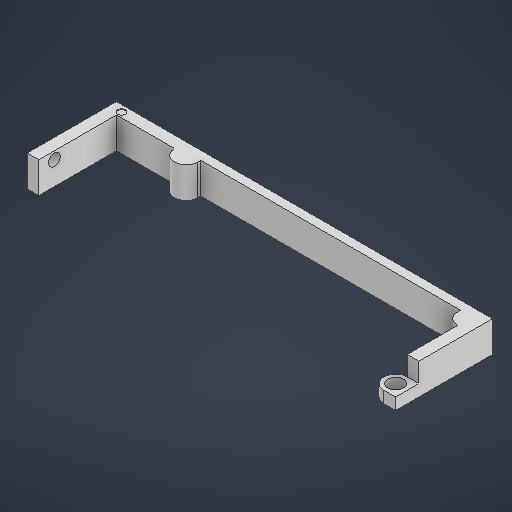
# Autodesk Inventor part: Część4
Saved by Autodesk Inventor 2026.2 (Build 302298010, 298A)
## iProperties
Created: 2026-04-27
Part Number: Część4
Material: Ogólny
Document SubType Name: Modeling
Designer: karol
Density: 1 g/cm^3
Appearance: Domyślna
Author: karol
Autodesk Inventor part; units mm, degrees
ref_plane "YZ Plane" through (0, 0, 0) normal (1, 0, 0) x (0, 1, 0)
ref_plane "XZ Plane" through (0, 0, 0) normal (0, 1, 0) x (-1, 0, 0)
ref_plane "XY Plane" through (0, 0, 0) normal (0, 0, 1) x (1, 0, 0)
sketch "Szkic1" plane through (0, 0, 0) normal (0, 1, 0) x (-1, 0, 0)
  line L0 (0, 0) -> (97, 0)
  line L1 (97, 0) -> (97, -3)
  line L2 (97, -3) -> (0, -3)
  line L3 (0, -3) -> (0, 0)
  dimension "d0" = 97
  dimension "d1" = 3
  constraints: 8 end point, 2 parallel, 1 horizontal, 1 perpendicular
  measures "d0" distance of L1.end L2.end
  measures "d1" distance of L0.end L1.end
extrude "Wyciągnięcie proste1" add sketch "Szkic1" along normal blind 8
sketch "Szkic2" plane through (0, 8, 0) normal (0, 1, 0) x (1, 0, 0)
  circle A0 centre (-94.0035, 1.3347) radius 1
  point P0 (0, 0)
  dimension "d4" = 2
  constraints: 1 centre point
  measures "d4" diameter of A0
extrude "Wyciągnięcie proste2" cut sketch "Szkic2" against normal blind 0.2
sketch "Szkic3" plane through (-97, 0, 0) normal (0, 0, 1) x (1, 0, 0)
  line L0 (97, 8) -> (0, 8) projected
  line L1 (97, 0) -> (94, 0)
  line L2 (94, 0) -> (94, 8)
  line L3 (94, 8) -> (97, 8)
  line L4 (97, 8) -> (97, 0)
  line L5 (0, 0) -> (3, 0)
  line L6 (3, 0) -> (3, 8)
  line L7 (3, 8) -> (0, 8)
  line L8 (0, 8) -> (0, 0)
  dimension "d7" = 3
  dimension "d8" = 3
  constraints: 16 end point, 4 parallel, 3 point on line, 2 horizontal, 2 perpendicular
  measures "d7" distance of L2.end L3.end
  measures "d8" distance of L7.end L6.end
extrude "Wyciągnięcie proste3" add sketch "Szkic3" along normal blind 20 contours L6 L5 L8 L0
extrude "Wyciągnięcie proste4" add sketch "Szkic3" along normal blind 19 contours L4 L1 L2 L0
sketch "Szkic4" plane through (-3, 0, 0) normal (-1, 0, 0) x (0, 0, 1)
  line L0 (19, 8) -> (19, 0) projected
  line L1 (0, 8) -> (19, 8) projected
  line L2 (19, 0) -> (14, 0)
  line L3 (14, 0) -> (14, 8)
  line L4 (14, 8) -> (19, 8)
  line L5 (19, 8) -> (19, 0)
  point P0 (0, 0)
  dimension "d13" = 5
  constraints: 8 end point, 2 parallel, 1 horizontal, 1 perpendicular, 1 point on line
  measures "d13" distance of L3.end L4.end
extrude "Wyciągnięcie proste5" add sketch "Szkic4" along normal blind 3
sketch "Szkic5" plane through (0, 8, 0) normal (0, 1, 0) x (1, 0, 0)
  line L0 (-94, 0) -> (-3, 0) projected
  line L1 (-3, 0) -> (-6, 0)
  line L2 (-6, 0) -> (-6, -3)
  line L3 (-6, -3) -> (-3, -3)
  line L4 (-3, -3) -> (-3, 0)
  line L5 (-79, 0) -> (-73, 0)
  line L6 (-73, 0) -> (-73, -3)
  line L7 (-73, -3) -> (-79, -3)
  line L8 (-79, -3) -> (-79, 0)
  line L9 (-3, 0) -> (-3, -14) projected
  point P0 (0, 0)
  dimension "d16" = 3
  dimension "d17" = 3
  dimension "d18" = 6
  dimension "d19" = 70
  dimension "d20" = 3
  constraints: 16 end point, 4 parallel, 2 horizontal, 2 perpendicular, 2 point on line
  measures "d16" distance of L3.end L2.end
  measures "d17" distance of L2.end L1.end
  measures "d18" distance of L6.end L7.end
  measures "d19" distance between parallel lines of L9 L6
  measures "d20" distance of L6.end L5.end
extrude "Wyciągnięcie proste6" add sketch "Szkic5" against normal blind 8
sketch "Szkic6" plane through (0, 8, 0) normal (0, 1, 0) x (1, 0, 0)
  line L0 (-3, -3) -> (-6, -3) projected
  line L1 (0, 3) -> (0, -19) projected
  line L2 (-6, -3) -> (0, 3)
  line L3 (0, -3) -> (-6, 3)
  line L4 (0, 3) -> (-97, 3) projected
  line L5 (-79, -3) -> (-79, 0) projected
  line L6 (-79, -3) -> (-73, 3)
  line L7 (-73, 3) -> (-73, -3)
  line L8 (-73, -3) -> (-79, 3)
  circle A0 centre (-76, 0) radius 2
  circle A1 centre (-3, 0) radius 2
  point P0 (0, 0)
  dimension "d23" = 4
  dimension "d24" = 4
  constraints: 10 end point, 3 point on line, 2 centre point, 2 midpoint, 2 perpendicular, 1 parallel
  measures "d23" diameter of A0
  measures "d24" diameter of A1
extrude "Wyciągnięcie proste7" cut sketch "Szkic6" against normal blind 8 contours A1 L3 L2 | L2 L3 A1 | A1 L2 L3 | L2 A1 L3 | A0 L8 L6 | L6 L8 A0 | L8 L6 A0 | L8 A0 L6
sketch "Szkic7" plane through (0, 8, 0) normal (0, 1, 0) x (1, 0, 0)
  circle A0 centre (-3, 0) radius 2 projected
  circle A1 centre (-3, 0) radius 2
  circle A2 centre (-76, 0) radius 2 projected
  circle A3 centre (-76, 0) radius 2
  point P0 (0, 0)
  constraints: 2 centre point, 2 coincident
extrude "Wyciągnięcie proste8" add sketch "Szkic7" against normal blind 3
sketch "Szkic8" plane through (-73, 0, 0) normal (0, 0, 1) x (1, 0, 0)
  line L0 (0, 8) -> (0, 0) projected
  line L1 (73, 8) -> (-24, 8) projected
  line L2 (0, 0) -> (13, 0)
  line L3 (13, 0) -> (13, 8)
  line L4 (13, 8) -> (0, 8)
  line L5 (0, 8) -> (0, 0)
  point P0 (73, 0)
  dimension "d29" = 13
  constraints: 8 end point, 2 parallel, 1 horizontal, 1 perpendicular, 1 point on line
  measures "d29" distance of L4.end L3.end
extrude "Wyciągnięcie proste9" cut sketch "Szkic8" against normal blind 0.5
sketch "Szkic10" plane through (-6, 0, 0) normal (0, 0, 1) x (1, 0, 0)
  line L0 (-54, 8) -> (-54, 0) projected
  line L1 (6, 8) -> (0, 8) projected
  line L2 (-54, 0) -> (0, 0)
  line L3 (0, 0) -> (0, 8)
  line L4 (0, 8) -> (-54, 8)
  line L5 (-54, 8) -> (-54, 0)
  point P0 (6, 0)
  constraints: 8 end point, 2 parallel, 1 horizontal, 1 perpendicular
extrude "Wyciągnięcie proste11" cut sketch "Szkic10" against normal blind 0.5
sketch "Szkic11" plane through (-73, 0, -0.5) normal (0, 0, 1) x (1, 0, 0)
  line L0 (0, 0) -> (0, 8) projected
  line L1 (67, 8) -> (67, 0) projected
  line L2 (0, 0) -> (67, 0)
  line L3 (67, 0) -> (67, 8)
  line L4 (67, 8) -> (0, 8)
  line L5 (0, 8) -> (0, 0)
  point P0 (73, 0)
  constraints: 8 end point, 2 parallel, 1 horizontal, 1 perpendicular
extrude "Wyciągnięcie proste12" add sketch "Szkic11" along normal blind 0.25
sketch "Szkic12" plane through (-73, 0, -0.25) normal (0, 0, 1) x (1, 0, 0)
  line L0 (67, 8) -> (67, 0) projected
  line L1 (0, 0) -> (0, 8) projected
  line L2 (67, 8) -> (0, 8)
  line L3 (0, 8) -> (0, 0)
  line L4 (0, 0) -> (67, 0)
  line L5 (67, 0) -> (67, 8)
  point P0 (73, 0)
  constraints: 8 end point, 2 parallel, 1 horizontal, 1 perpendicular
extrude "Wyciągnięcie proste13" cut sketch "Szkic12" against normal blind 0.5
sketch "Szkic13" plane through (-97, 0, -3) normal (-1, 0, 0) x (0, 0, 1)
  circle A0 centre (19, 6) radius 1.5
  line L0 (0, 8) -> (23, 8) projected
  line L1 (23, 8) -> (23, 0) projected
  point P0 (3, 0)
  dimension "d40" = 3
  dimension "d41" = 2
  dimension "d42" = 4
  constraints: 1 centre point
  measures "d40" diameter of A0
  measures "d41" distance from line of L0 A0.centre
  measures "d42" distance from line of L1 A0.centre
extrude "Wyciągnięcie proste14" cut sketch "Szkic13" against normal up to surface (3 mm away)
sketch "Szkic14" plane through (0, 8, 0) normal (0, 1, 0) x (1, 0, 0)
  line L0 (-3, -14) -> (-6, -14) projected
  line L1 (0, -19) -> (-6, -19) projected
  line L2 (-3, -14) -> (-6, -14)
  line L3 (-6, -14) -> (-6, -19)
  line L4 (-6, -19) -> (-3, -19)
  line L5 (-3, -19) -> (-3, -14)
  line L6 (0, -19) -> (-3, -19)
  line L7 (-3, -19) -> (-3, -16)
  line L8 (-3, -16) -> (0, -16)
  line L9 (0, -16) -> (0, -19)
  point P0 (0, 0)
  dimension "d45" = 3
  dimension "d46" = 3
  constraints: 16 end point, 4 parallel, 2 horizontal, 2 perpendicular
  measures "d45" distance of L7.end L8.end
  measures "d46" distance of L6.end L7.end
extrude "Wyciągnięcie proste15" cut sketch "Szkic14" against normal blind 8
sketch "Szkic15" plane through (0, 0, 0) normal (0, -1, 0) x (1, 0, 0)
  line L0 (0, 16) -> (-3, 16) projected
  line L1 (0, 16) -> (-6, 16)
  line L2 (-6, 16) -> (-6, 22)
  line L3 (-6, 22) -> (0, 22)
  line L4 (0, 22) -> (0, 16)
  point P0 (0, 0)
  dimension "d49" = 6
  dimension "d50" = 6
  constraints: 8 end point, 2 parallel, 1 horizontal, 1 perpendicular
  measures "d49" distance of L2.end L3.end
  measures "d50" distance of L1.end L2.end
extrude "Wyciągnięcie proste16" add sketch "Szkic15" against normal blind 3
sketch "Szkic17" plane through (0, 0, 0) normal (0, -1, 0) x (1, 0, 0)
  circle A0 centre (-3, 19) radius 2
  line L0 (0, -3) -> (0, 22) projected
  line L1 (0, 22) -> (-6, 22) projected
  point P0 (0, 0)
  point P1 (-3, 22)
  dimension "d53" = 4
  dimension "d54" = 3
  dimension "d55" = 3
  constraints: 1 centre point, 1 midpoint
  measures "d53" diameter of A0
  measures "d54" distance from line of L0 A0.centre
  measures "d55" distance of point (-3, 22) A0.centre
extrude "Wyciągnięcie proste17" cut sketch "Szkic17" against normal blind 3
fillet "Fillet1" radius 3 2 edges at (-73, 4, 3) (-79, 4, 3)
fillet "Fillet2" radius 3 1 edges at (-6, 4, 3)
fillet "Fillet3" radius 3 2 edges at (-6, 1.5, 22) (-6, 1.5, 16)
